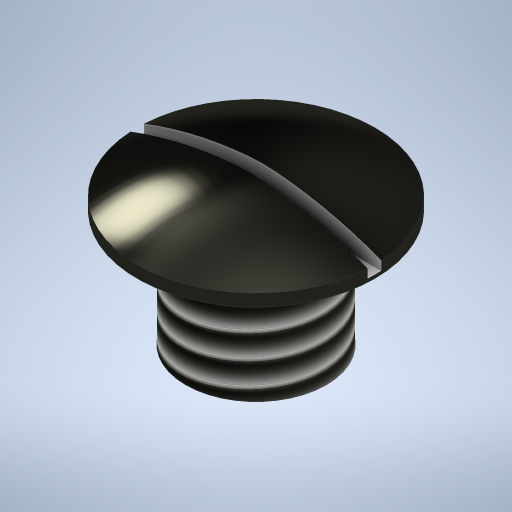
# Autodesk Inventor part: prafuso3
Saved by Autodesk Inventor 2023 (Build 270158000, 158)
## iProperties
Created: 2023-08-09
Part Number: prafuso3
Material: Genérico
Document SubType Name: Modeling
Designer: azeve
Density: 1 g/cm^3
Appearance: Padrão
Author: azeve
Autodesk Inventor part; units mm, degrees
ref_plane "YZ Plane" through (0, 0, 0) normal (1, 0, 0) x (0, 1, 0)
sketch "Esboço1" plane through (0, 0, 0) normal (0, 0, 1) x (1, 0, 0)
  line L0 (0, 0) -> (1.45, 0)
  line L1 (1.45, 0) -> (1.45, 2.4)
  line L2 (1.45, 2.4) -> (2.45, 2.4)
  line L3 (2.45, 2.4) -> (8.95, 2.4)
  line L4 (2.45, 2.4) -> (2.45, 2.65)
  line L5 (0, 0) -> (0, 3.1668)
  line L6 (1.45, 0) -> (0, 0)
  arc A0 (2.45, 2.65) -> (0, 3.1668) centre (-0.3817, -4.7083) ccw
  point P0 (0, 2.5981)
  dimension "d0" = 1.45
  dimension "d1" = 2.4
  dimension "d11" = 1
  constraints: 14 end point, 2 horizontal, 2 point on circle, 2 point on line, 2 vertical, 1 centre point, 1 collinear, 1 perpendicular
  measures "d0" distance of L0.start L0.end
  measures "d1" distance of L0.end L1.end
  measures "d11" distance of L1.end L2.end
revolve "Revolução1" add sketch "Esboço1" angle 360 about axis through (0, 0, 0) along (0, 1, 0)
thread "Rosca1" size "M30x3.5" class "6g" standard "ANSI Metric M Profile" full length
ref_plane "Plano de trabalho1" through (0, 14.65, 0) normal (0, -1, 0) x (1, 0, 0)
sketch "Esboço2" plane through (0, 14.65, 0) normal (0, -1, 0) x (1, 0, 0)
  line L0 (23.8734, 2.4868) -> (-23.8734, 2.4868)
  line L1 (-23.8734, 2.4868) -> (-23.8734, -2.4868)
  line L2 (-23.8734, -2.4868) -> (23.8734, -2.4868)
  line L3 (23.8734, -2.4868) -> (23.8734, 2.4868)
  line L4 (23.8734, 2.4868) -> (-23.8734, -2.4868) construction
  line L5 (-23.8734, 2.4868) -> (23.8734, -2.4868) construction
  point P0 (0, 0)
  constraints: 12 end point, 2 midpoint, 2 parallel, 1 horizontal, 1 perpendicular
extrude "Extrusão1" cut sketch "Esboço2" along normal blind 11
thread "Rosca2" size "M3x0.5" class "6g" standard "ANSI Metric M Profile" full length
ref_plane "Plano de trabalho2" through (0, 3.4, 0) normal (0, -1, 0) x (1, 0, 0)
sketch "Esboço3" plane through (0, 3.4, 0) normal (0, -1, 0) x (1, 0, 0)
  line L0 (-2.7014, -0.145) -> (2.7014, -0.145)
  line L1 (2.7014, -0.145) -> (2.7014, 0.145)
  line L2 (2.7014, 0.145) -> (-2.7014, 0.145)
  line L3 (-2.7014, 0.145) -> (-2.7014, -0.145)
  line L4 (-2.7014, -0.145) -> (2.7014, 0.145) construction
  line L5 (2.7014, -0.145) -> (-2.7014, 0.145) construction
  point P0 (0, 0)
  constraints: 12 end point, 2 midpoint, 2 parallel, 1 horizontal, 1 perpendicular
extrude "Extrusão2" cut sketch "Esboço3" along normal blind 0.93
